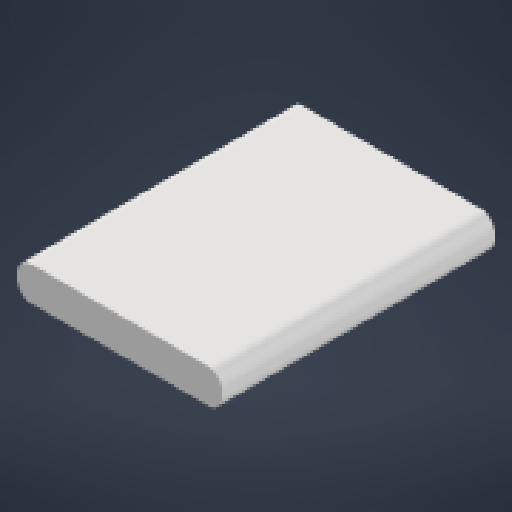
# Autodesk Inventor part: Battery_atrapa
Saved by Autodesk Inventor 2024.4 (Build 284460000, 460)
## iProperties
Created: 2026-03-15
Part Number: Battery_atrapa
Material: Ogólny
Document SubType Name: Modeling
Designer: User
Density: 1 g/cm^3
Appearance: Domyślna
Author: User
Autodesk Inventor part; units mm, degrees
ref_plane "YZ Plane" through (0, 0, 0) normal (1, 0, 0) x (0, 1, 0)
ref_plane "XZ Plane" through (0, 0, 0) normal (0, 1, 0) x (-1, 0, 0)
ref_plane "XY Plane" through (0, 0, 0) normal (0, 0, 1) x (1, 0, 0)
sketch "Szkic1" plane through (0, 0, 0) normal (0, 1, 0) x (-1, 0, 0)
  line L0 (-15, 20) -> (15, 20)
  line L1 (15, 20) -> (15, -20)
  line L2 (15, -20) -> (-15, -20)
  line L3 (-15, -20) -> (-15, 20)
  line L4 (-15, 20) -> (15, -20) construction
  line L5 (15, 20) -> (-15, -20) construction
  point P0 (0, 0)
  dimension "d0" = 30
  dimension "d1" = 40
  constraints: 12 end point, 2 midpoint, 2 parallel, 1 horizontal, 1 perpendicular
  measures "d0" distance of L1.end L2.end
  measures "d1" distance of L0.end L1.end
extrude "Wyciągnięcie proste1" add sketch "Szkic1" along normal blind 5
fillet "Zaokrąglenie1" radius 2 4 edges at (15, 5, 0) (-15, 5, 0) (15, 0, 0) (-15, 0, 0)
